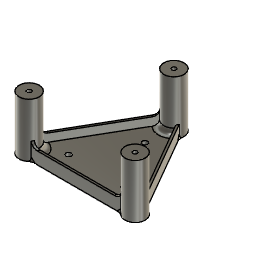
stevenson_spacer_bottom v5 (Autodesk Fusion 360 design; units mm, degrees)
Autodesk Fusion 360 part; units mm, degrees
sketch "Sketch1" plane through (0, 0, 0) normal (0, 0, 1) x (1, 0, 0)
  circle A0 centre (0, 0) radius 60 construction
  circle A1 centre (0, 0) radius 22.5 construction
  circle A2 centre (0, 0) radius 45.5 construction
  circle A3 centre (0, 45.5) radius 4.5
  circle A4 centre (-39.4042, -22.75) radius 4.5
  circle A5 centre (39.4042, -22.75) radius 4.5
  line L0 (0, 0) -> (0, 45.5) construction
  line L1 (0, 0) -> (39.4042, -22.75) construction
  line L2 (0, 0) -> (-39.4042, -22.75) construction
  circle A6 centre (-39.4042, -22.75) radius 2
  circle A7 centre (39.4042, -22.75) radius 2
  circle A8 centre (0, 45.5) radius 2
  line L3 (-43.3013, -20.5) -> (-3.8971, 47.75)
  line L4 (-39.4042, -27.25) -> (39.4042, -27.25)
  line L5 (3.8971, 47.75) -> (43.3013, -20.5)
  line L6 (-38.5819, -18.3258) -> (-3.4204, 42.5758)
  line L7 (3.4204, 42.5758) -> (38.5819, -18.3258)
  line L8 (-35.1615, -24.25) -> (35.1615, -24.25)
  dimension "d5" = 120
  dimension "d7" = 45
  dimension "d10" = 91
  dimension "d12" = 9
  dimension "d13" = 120
  dimension "d14" = 120
  dimension "d16" = 4
  dimension "d19" = 3
  dimension "d20" = 3
  dimension "d21" = 3
  constraint coincident A0.centre A1.centre
  constraint concentric A1 A2
  constraint coincident A2 A3.centre
  constraint coincident A2 A4.centre
  constraint coincident A2 A5.centre
  constraint equal A3 A5
  constraint equal A4 A5
  constraint coincident A3.centre L0.end
  constraint coincident A5.centre L1.end
  constraint coincident A4.centre L2.end
  constraint vertical A0.centre A3.centre
  constraint concentric A4 A6
  constraint concentric A5 A7
  constraint equal A7 A8
  constraint equal A6 A7
  constraint coincident A4 L3.start
  constraint coincident A3 L3.end
  constraint coincident A4 L4.start
  constraint coincident A5 L4.end
  constraint horizontal L4
  constraint coincident A3 L5.start
  constraint coincident A5 L5.end
  constraint equal L3 L5
  constraint equal L4 L5
  constraint tangent A3 L3
  constraint tangent A4 L3
  constraint tangent A5 L4
  constraint tangent A5 L5
  constraint coincident A4 L6.start
  constraint coincident A3 L6.end
  constraint coincident A3 L7.start
  constraint coincident A5 L7.end
  constraint coincident A4 L8.start
  constraint coincident A5 L8.end
  constraint horizontal L8
  constraint parallel L3 L6
  constraint parallel L5 L7
  measures "d5" diameter of A0
  measures "d7" diameter of A1
  measures "d10" diameter of A2
  measures "d12" diameter of A3
  measures "d13" angle of L0 L1
  measures "d14" angle of L1 L2
  measures "d16" diameter of A8
  measures "d19" distance of L3 L6
  measures "d20" distance of L4 L8
  measures "d21" distance of L5 L7
extrude "Extrude1" add sketch "Sketch1" along normal blind 3 makes body 1
extrude "Extrude2" add sketch "Sketch1" along normal blind 40 contours A3 | A5 | A4 bodies 1
sketch "Sketch3" plane through (0, 0, 40) normal (0, 0, 1) x (-1, 0, 0)
  circle A0 centre (39.4042, 22.75) radius 2
  circle A1 centre (39.4042, 22.75) radius 4.5
  circle A2 centre (39.4042, 22.75) radius 2.5
  circle A3 centre (-39.4042, 22.75) radius 2.5
  circle A4 centre (0, -45.5) radius 2.5
  dimension "d29" = 5
  dimension "d31" = 360
  constraint concentric A0 A2
  measures "d29" diameter of A2
extrude "Extrude3" cut sketch "Sketch3" against normal blind 5 contours A2 | A3 | A4 bodies 1
fillet "Fillet1" [no effect]
fillet "Fillet2" radius 5 3 edges at (35.507, -20.5, 3) (-35.507, -20.5, 3) (0, 41, 3) on bodies 1
sketch "Sketch5" plane through (0, 0, 0) normal (1, 0, 0) x (0, 1, 0)
  line L0 (60, 0) -> (-60, 0) construction
  line L1 (60, 40) -> (51.4977, 0)
  line L2 (51.4977, 0) -> (48.4307, 0)
  line L3 (48.4307, 0) -> (56.933, 40)
  line L4 (56.933, 40) -> (60, 40)
  line L5 (50, 40) -> (41, 40) construction
  line L6 (60, 40) -> (60, 0) construction
  dimension "d39" = 12
  dimension "d40" = 3
  constraint coincident L0 L1.end
  constraint coincident L0 L2.end
  constraint parallel L1 L3
  constraint parallel L0 L4
  constraint horizontal L3.end L5.start
  constraint vertical L0.start L1.start
  constraint coincident L0.start L6.end
  measures "d39" angle of L1 L6
  measures "d40" distance of L1 L3
revolve "Revolve1" add sketch "Sketch5" angle 360 about axis through (0, 0, 1.75) along (0, 0, 1) separate body makes body 2
sketch "Sketch7" plane through (0, 0, 40) normal (0, 0, 1) x (-1, 0, 0)
  circle A0 centre (0, 0) radius 56.933
  circle A1 centre (0, 0) radius 60
  line L0 (0, 0) -> (-30, -51.9615) construction
  line L1 (-23.7213, -55.5865) -> (-36.2787, -48.3365)
  line L2 (-36.2787, -48.3365) -> (-30.2212, -37.8446)
  line L3 (-30.2212, -37.8446) -> (-17.6638, -45.0946)
  line L4 (-17.6638, -45.0946) -> (-23.7213, -55.5865)
  circle A2 centre (0, 0) radius 48.4307 construction
  line L5 (0, 0) -> (0, -48.4307) construction
  dimension "d44" = 14.5
  dimension "d46" = 30
  constraint coincident A0.centre A1.centre
  constraint coincident A1 L0.end
  constraint midpoint L0.end L1
  constraint coincident L2.end A2
  constraint perpendicular L0 L1
  constraint perpendicular L1 L4
  constraint perpendicular L3 L4
  constraint perpendicular L2 L3
  constraint coincident A2 L5.end
  constraint vertical L5
  measures "d44" distance of L1.start L1.end
  measures "d46" angle of L0 L5
extrude "Extrude4" cut sketch "Sketch7" against normal blind 5.7 contours A0 L2 L3 L4 | A0 A1 L2 L4 picked at (-26.1412, -43.6629) picked at (-28.9605, -50.161) bodies 2
pattern_circular "C-Pattern1" count 6 over 360 about axis through (0, 0, 1.75) along (0, 0, 1) of "Extrude4"
chamfer "Chamfer2" distance 3.5 angle 45 12 edges at (-22.1182, 52.8098, 34.3) (22.1182, 52.8098, 34.3) (56.7937, 7.25, 34.3) (-56.7937, 7.25, 34.3) (-34.6755, -45.5598, 34.3) (34.6755, -45.5598, 34.3) (56.7937, -7.25, 34.3) (22.1182, -52.8098, 34.3) (-56.7937, -7.25, 34.3) (-34.6755, 45.5598, 34.3) (34.6755, 45.5598, 34.3) (-22.1182, -52.8098, 34.3) on bodies 2
sketch "Sketch8" plane through (0, 0, 0) normal (1, 0, 0) x (0, 1, 0)
  line L0 (90, 55) -> (-90, 55)
  line L1 (-90, 55) -> (-90, -30)
  line L2 (-90, -30) -> (90, -30)
  line L3 (90, -30) -> (90, 55)
  constraint horizontal L0
  constraint vertical L1
  constraint horizontal L2
  constraint vertical L3
sketch "Sketch9" plane through (0, 0, 0) normal (0, 0, -1) x (1, 0, 0)
  circle A0 centre (39.4042, 22.75) radius 2
  circle A1 centre (-39.4042, 22.75) radius 2
  arc A2 (43.3013, 20.5) -> (39.4042, 27.25) centre (39.4042, 22.75) ccw
  line L0 (39.4042, 27.25) -> (-39.4042, 27.25)
  arc A3 (-39.4042, 27.25) -> (-43.3013, 20.5) centre (-39.4042, 22.75) ccw
  line L1 (-43.3013, 20.5) -> (-3.8971, -47.75)
  arc A4 (-3.8971, -47.75) -> (3.8971, -47.75) centre (0, -45.5) ccw
  line L2 (3.8971, -47.75) -> (43.3013, 20.5)
  circle A5 centre (0, -45.5) radius 2
  circle A6 centre (0, -45.5) radius 2.5
  circle A7 centre (-39.4042, 22.75) radius 2.5
  circle A8 centre (39.4042, 22.75) radius 2.5
  dimension "d56" = 5
  constraint concentric A4 A6
  constraint concentric A1 A7
  constraint concentric A0 A8
  constraint equal A6 A7
  constraint equal A6 A8
  measures "d56" diameter of A6
extrude "Extrude6" cut sketch "Sketch9" against normal up to surface (33 mm away) contours A6 | A7 | A8 bodies 1
chamfer "Chamfer3" distance 0.5 angle 45 3 edges at (-41.735, -21.846, 33) (-2.3308, 46.404, 33) (37.0733, -21.846, 33) on bodies 1
sketch "Sketch10" plane through (0, 0, 40) normal (0, 0, 1) x (-1, 0, 0)
  circle A0 centre (0, -45.5) radius 2.5
  circle A1 centre (0, -45.5) radius 4.5
  arc A2 (-21.9561, -52.529) -> (21.9561, -52.529) centre (0, 0) ccw
  circle A3 centre (0, -45.5) radius 4.5
  circle A4 centre (0, -45.5) radius 2.5
  line L0 (21.9561, -52.529) -> (13.8983, -38.5725)
  line L1 (-21.9561, -52.529) -> (-13.8983, -38.5725)
  arc A5 (-13.8983, -38.5725) -> (13.8983, -38.5725) centre (0, 0) ccw
  line L2 (19.8231, -51.2316) -> (13.7644, -40.7375)
  line L3 (-19.8231, -51.2316) -> (-13.7644, -40.7375)
  arc A6 (-19.8231, -51.2316) -> (19.8231, -51.2316) centre (0, 0) ccw
  arc A7 (-5.8194, -42.6044) -> (5.8194, -42.6044) centre (0, -45.5) ccw
  arc A8 (-13.7644, -40.7375) -> (-5.8194, -42.6044) centre (0, 0) ccw
  arc A9 (5.8194, -42.6044) -> (13.7644, -40.7375) centre (0, 0) ccw
  arc A10 (-31.0451, -46.2717) -> (-24.5499, -50.0217) centre (0, 0) ccw construction
  arc A11 (24.5499, -50.0217) -> (31.0451, -46.2717) centre (0, 0) ccw construction
  line L4 (-27.8607, -48.2562) -> (0, 0) construction
  line L5 (0, 0) -> (27.8607, -48.2562) construction
  line L6 (0, -52) -> (0, -54.933) construction
  line L7 (1.0754, -51.9104) -> (1.0754, -54.9225)
  line L8 (-1.0754, -51.9104) -> (-1.0754, -54.9225)
  dimension "d70" = 2.1508
  constraint coincident A2.end L0.start
  constraint coincident A2.start L1.start
  constraint coincident L0.end A5.end
  constraint tangent A1 A5
  constraint concentric A1 A7
  constraint coincident A7.end A8
  constraint parallel L0 L2
  constraint concentric A5 A8
  constraint parallel L1 L3
  constraint concentric A2 A6
  constraint concentric A8 A9
  constraint midpoint A10 L4.start
  constraint coincident A2.centre A5.centre
  constraint midpoint A11 L5.end
  constraint parallel L0 L5
  constraint parallel L1 L4
  constraint midpoint A7 L6.start
  constraint midpoint A6 L6.end
  constraint vertical L6
  constraint coincident A7 L7.start
  constraint coincident A6 L7.end
  constraint vertical L7
  constraint coincident A7 L8.start
  constraint coincident A6 L8.end
  constraint parallel L6 L8
  constraint equal L7 L8
  measures "d70" distance of L7 L8
extrude "Extrude7" add sketch "Sketch10" against normal blind 1.2 contours A1 A3 | A2 L0 L1 A5 | A6 A7 L7 L8 bodies 2
pattern_circular "C-Pattern2" count 6 over 360 about axis through (0, 0, 1.75) along (0, 0, 1) of "Extrude7"
sketch "Sketch11" plane through (0, 0, 0) normal (0, 0, 1) x (1, 0, 0)
  circle A0 centre (0, 0) radius 68.9895
  constraint coincident A0.centre origin
extrude "Extrude8" cut sketch "Sketch11" along normal up to surface (31.9 mm away) bodies 2
sketch "Sketch12" plane through (0, 0, 0) normal (1, 0, 0) x (0, 1, 0)
  line L0 (50, 40) -> (41, 40) construction
  line L1 (50, 0) -> (47.75, 0) construction
  line L2 (50, 40) -> (50, 0)
  line L3 (50, 40) -> (53, 40)
  line L4 (53, 40) -> (50, 35.7156)
  line L5 (50, 4.2844) -> (53, 0)
  line L6 (53, 0) -> (50, 0)
  dimension "d71" = 35
  dimension "d72" = 35
  dimension "d73" = 3
  constraint coincident L0.start L2.start
  constraint coincident L1.start L2.end
  constraint perpendicular L2 L3
  constraint coincident L2 L4.end
  constraint coincident L2 L5.start
  constraint perpendicular L2 L6
  constraint equal L3 L6
  measures "d71" angle of L2 L4
  measures "d72" angle of L2 L5
  measures "d73" distance of L0.start L3.end
revolve "Revolve2" add sketch "Sketch12" angle 360 about axis through (0, 45.5, 40) along (0, 0, 1) bodies 1
fillet "Fillet3" radius 4 3 edges at (5.1962, 45.5, 3.2902) (0, 50, 4.2844) (-5.1962, 45.5, 3.2902) on bodies 1
pattern_circular "C-Pattern3" count 3 over 360 about axis through (0, 0, 1.75) along (0, 0, 1) of "Revolve2", "Fillet3"
sketch "Sketch14" plane through (0, 0, 40) normal (0, 0, 1) x (-1, 0, 0)
  circle A0 centre (0, -45.5) radius 7.5
  circle A1 centre (0, -45.5) radius 2.5
  circle A2 centre (0, -45.5) radius 2.5
  line L0 (2, -47) -> (-2, -47)
  dimension "d80" = 4
  constraint coincident A2 L0.start
  constraint coincident A2 L0.end
  constraint horizontal L0
  measures "d80" distance of L0.start L0.end
extrude "Extrude9" add sketch "Sketch14" against normal up to surface (40 mm away) contours A1 A2 L0 picked at (-0.6667, -47.4632) bodies 1
pattern_circular "C-Pattern4" count 3 over 360 about axis through (0, 0, 1.75) along (0, 0, 1) of "Extrude9"
ref_plane "WorkPlane1" through (0, 45.5, 45) normal (0, 0, 1) x (1, 0, 0)
sketch "Sketch15" plane through (0, 45.5, 45) normal (0, 0, 1) x (1, 0, 0)
  arc A0 (-2, 1.5) -> (2, 1.5) centre (0, 0) ccw
  line L0 (-2, 1.5) -> (2, 1.5)
  arc A1 (-1.8974, 1.3) -> (1.8974, 1.3) centre (0, 0) ccw
  line L1 (-1.8974, 1.3) -> (1.8974, 1.3)
  dimension "d88" = 0.2
extrude "Extrude10" add sketch "Sketch15" along normal blind 15 separate body contours A1 L1 makes body 3
sketch "Sketch16" plane through (0, 0, 40) normal (0, 0, 1) x (-1, 0, 0)
  circle A0 centre (0, -45.5) radius 7.5
  arc A1 (2, -47) -> (-2, -47) centre (0, -45.5) ccw
  line L0 (2, -47) -> (-2, -47)
extrude "Extrude11" add sketch "Sketch16" 2 faces at (-42.4352, -24.5, 40) (42.4352, -24.5, 40) along normal up to surface end surface through (7.4268, 44.4549, 0) normal (0, 0, 1) offset 0 on bodies 1 bodies 1
fillet "Fillet4" radius 4 2 edges at (0, 38, 3.4174) (0, 38, 3.4174) on bodies 1
fillet "Fillet4" radius 4 4 edges at (-32.909, -19, 3.4174) (-32.909, -19, 3.4174) (32.909, -19, 3.4174) (32.909, -19, 3.4174) on bodies 1
sketch "Sketch17" plane through (0, 0, 3) normal (0, 0, 1) x (-1, 0, 0)
  arc A0 (-38.0098, 11.3348) -> (-28.8212, 27.25) centre (-39.4042, 22.75) ccw
  line L0 (-38.0098, 11.3348) -> (-9.1886, -38.5848)
  arc A1 (9.1886, -38.5848) -> (-9.1886, -38.5848) centre (0, -45.5) ccw
  line L1 (9.1886, -38.5848) -> (38.0098, 11.3348)
  arc A2 (28.8212, 27.25) -> (38.0098, 11.3348) centre (39.4042, 22.75) ccw
  line L2 (28.8212, 27.25) -> (-28.8212, 27.25)
  circle A3 centre (0, -24) radius 2
  circle A4 centre (20.7846, 12) radius 2
  circle A5 centre (-20.7846, 12) radius 2
  point P0 (0, -34)
  dimension "d97" = 4
  dimension "d98" = 10
  dimension "d100" = 360
  constraint midpoint A1 P0
  constraint vertical origin A3.centre
  measures "d97" diameter of A3
  measures "d98" distance of A3.centre P0
extrude "Extrude12" cut sketch "Sketch17" against normal up to surface (3 mm away) contours A3 | A4 | A5 bodies 1
sketch "Sketch18" plane through (0, 0, 3) normal (0, 0, 1) x (-1, 0, 0)
  circle A0 centre (20.7846, 12) radius 2
  circle A1 centre (0, -24) radius 2
  circle A2 centre (-20.7846, 12) radius 2
  arc A3 (-38.0098, 11.3348) -> (-28.8212, 27.25) centre (-39.4042, 22.75) ccw
  line L0 (-38.0098, 11.3348) -> (-9.1886, -38.5848)
  arc A4 (9.1886, -38.5848) -> (-9.1886, -38.5848) centre (0, -45.5) ccw
  line L1 (9.1886, -38.5848) -> (38.0098, 11.3348)
  arc A5 (28.8212, 27.25) -> (38.0098, 11.3348) centre (39.4042, 22.75) ccw
  line L2 (28.8212, 27.25) -> (-28.8212, 27.25)
  line L3 (35, 25.65) -> (-34.8846, 25.65)
  line L4 (-34.8846, 25.65) -> (-35.6422, 27.25)
  line L5 (-35.6422, 27.25) -> (35, 27.25)
  line L6 (35, 27.25) -> (35, 25.65)
  line L7 (-39.7136, 17.4859) -> (-4.7713, -43.0359)
  line L8 (-5.7781, -44.492) -> (-41.0992, 16.6859)
  line L9 (-41.0992, 16.6859) -> (-39.7136, 17.4859)
  line L10 (-4.7713, -43.0359) -> (-5.7781, -44.492)
  line L11 (4.7136, -43.1359) -> (39.6558, 17.3859)
  line L12 (41.4203, 17.242) -> (6.0992, -43.9359)
  line L13 (6.0992, -43.9359) -> (4.7136, -43.1359)
  line L14 (39.6558, 17.3859) -> (41.4203, 17.242)
  dimension "d103" = 1.6
  dimension "d105" = 360
  constraint parallel L2 L3
  constraint parallel L2 L5
  constraint perpendicular L5 L6
  constraint collinear L2 L5
  measures "d103" distance of L3 L5
extrude "Extrude13" add sketch "Sketch18" along normal blind 6 contours A3 L7 L8 L9 | A3 L0 A4 L7 L8 | A4 L7 L8 L10 | A3 L3 L4 L5 | A3 A5 L2 L3 L5 | A5 L3 L5 L6 | A4 L1 A5 L11 L12 | A4 L11 L12 L13 | A5 L11 L12 L14 bodies 1
fillet "Fillet5" radius 4 5 edges at (-6.4826, 41.7283, 9) (-39.3791, -15.25, 9) (-32.8965, -26.4783, 9) (39.3791, -15.25, 9) (32.8965, -26.4783, 9) on bodies 1
sketch "Sketch19" plane through (0, 0, 0) normal (0, 0, -1) x (1, 0, 0)
  circle A0 centre (-20.7846, 12) radius 2
  circle A1 centre (0, -24) radius 2
  circle A2 centre (20.7846, 12) radius 2
  arc A3 (39.7032, 25.2321) -> (41.7032, 21.7679) centre (39.4042, 22.75) ccw
  line L0 (39.7032, 25.2321) -> (41.7032, 21.7679)
  spline S0 degree 3 poles (30.3991, 27.25) (31.2433, 27.25) (32.0954, 27.3887) (33.6181, 27.9075) (34.264, 28.2527) (34.7938, 28.6656) knots 0 0 0 0 0.253267 0.253267 0.483496 0.483496 0.483496 0.483496
  line L1 (30.3991, 27.25) -> (-30.3991, 27.25)
  spline S1 degree 3 poles (-34.7938, 28.6656) (-34.2696, 28.2571) (-33.6317, 27.9148) (-32.1116, 27.3913) (-31.2513, 27.25) (-30.3991, 27.25) knots 0 0 0 0 0.19935 0.19935 0.423274 0.423274 0.423274 0.423274
  arc A4 (-34.7938, 28.6656) -> (-42.222, 15.7995) centre (-39.4042, 22.75) ccw
  spline S2 degree 3 poles (-38.7987, 12.7014) (-39.2216, 13.4338) (-39.7689, 14.1035) (-40.9801, 15.1619) (-41.6008, 15.5476) (-42.222, 15.7995) knots 0 0 0 0 0.253712 0.253712 0.483453 0.483453 0.483453 0.483453
  line L2 (-38.7987, 12.7014) -> (-8.3996, -39.9514)
  spline S3 degree 3 poles (-7.4283, -44.4651) (-7.3365, -43.8062) (-7.3591, -43.0817) (-7.6664, -41.5035) (-7.974, -40.6887) (-8.3996, -39.9514) knots 0 0 0 0 0.199576 0.199576 0.423259 0.423259 0.423259 0.423259
  arc A5 (-7.4283, -44.4651) -> (7.4283, -44.4651) centre (0, -45.5) ccw
  spline S4 degree 3 poles (8.3996, -39.9514) (7.9768, -40.6838) (7.6705, -41.4926) (7.3595, -43.0707) (7.3358, -43.8012) (7.4283, -44.4651) knots 0 0 0 0 0.253712 0.253712 0.483453 0.483453 0.483453 0.483453
  line L3 (8.3996, -39.9514) -> (38.7987, 12.7014)
  spline S5 degree 3 poles (42.222, 15.7995) (41.6055, 15.5495) (40.9894, 15.1676) (39.7763, 14.1125) (39.2244, 13.4387) (38.7987, 12.7014) knots 0 0 0 0 0.199576 0.199576 0.423259 0.423259 0.423259 0.423259
  arc A6 (42.222, 15.7995) -> (34.7938, 28.6656) centre (39.4042, 22.75) ccw
  arc A7 (2, -47) -> (-2, -47) centre (0, -45.5) ccw
  line L4 (2, -47) -> (-2, -47)
  arc A8 (-41.7032, 21.7679) -> (-39.7032, 25.2321) centre (-39.4042, 22.75) ccw
  line L5 (-41.7032, 21.7679) -> (-39.7032, 25.2321)
  circle A9 centre (39.4042, 22.75) radius 1.4
  circle A10 centre (0, -45.5) radius 1.4
  circle A11 centre (-39.4042, 22.75) radius 1.4
  dimension "d111" = 2.8
  constraint concentric A3 A9
  constraint concentric A5 A10
  constraint concentric A4 A11
  constraint equal A9 A11
  constraint equal A9 A10
  measures "d111" diameter of A11
extrude "Extrude14" add sketch "Sketch19" against normal up to surface (32.5001 mm away) contours A3 L0 | A7 L4 | A8 L5 bodies 1
chamfer "Chamfer4" distance 0.4 distance2 3 3 edges at (-40.7094, -23.2563, 0) (38.0989, -23.2563, 0) (-1.3053, 44.9937, 0) measured on face at (-0.0498, 0.0863, 0) measured on face at (-0.0498, 0.0863, 0) measured on face at (-0.0498, 0.0863, 0) on bodies 1
sketch "Sketch20" plane through (0, 0, 0) normal (0, 0, -1) x (1, 0, 0)
  circle A0 centre (39.4042, 22.75) radius 1.8
  spline S0 degree 3 poles (30.3991, 27.25) (31.2433, 27.25) (32.0954, 27.3887) (33.6181, 27.9075) (34.264, 28.2527) (34.7938, 28.6656) knots 0 0 0 0 0.253267 0.253267 0.483496 0.483496 0.483496 0.483496
  line L0 (30.3991, 27.25) -> (-30.3991, 27.25)
  spline S1 degree 3 poles (-34.7938, 28.6656) (-34.2696, 28.2571) (-33.6317, 27.9148) (-32.1116, 27.3913) (-31.2513, 27.25) (-30.3991, 27.25) knots 0 0 0 0 0.19935 0.19935 0.423274 0.423274 0.423274 0.423274
  arc A1 (-34.7938, 28.6656) -> (-42.222, 15.7995) centre (-39.4042, 22.75) ccw
  spline S2 degree 3 poles (-38.7987, 12.7014) (-39.2216, 13.4338) (-39.7689, 14.1035) (-40.9801, 15.1619) (-41.6008, 15.5476) (-42.222, 15.7995) knots 0 0 0 0 0.253712 0.253712 0.483453 0.483453 0.483453 0.483453
  line L1 (-38.7987, 12.7014) -> (-8.3996, -39.9514)
  spline S3 degree 3 poles (-7.4283, -44.4651) (-7.3365, -43.8062) (-7.3591, -43.0817) (-7.6664, -41.5035) (-7.974, -40.6887) (-8.3996, -39.9514) knots 0 0 0 0 0.199576 0.199576 0.423259 0.423259 0.423259 0.423259
  arc A2 (-7.4283, -44.4651) -> (7.4283, -44.4651) centre (0, -45.5) ccw
  spline S4 degree 3 poles (8.3996, -39.9514) (7.9768, -40.6838) (7.6705, -41.4926) (7.3595, -43.0707) (7.3358, -43.8012) (7.4283, -44.4651) knots 0 0 0 0 0.253712 0.253712 0.483453 0.483453 0.483453 0.483453
  line L2 (8.3996, -39.9514) -> (38.7987, 12.7014)
  spline S5 degree 3 poles (42.222, 15.7995) (41.6055, 15.5495) (40.9894, 15.1676) (39.7763, 14.1125) (39.2244, 13.4387) (38.7987, 12.7014) knots 0 0 0 0 0.199576 0.199576 0.423259 0.423259 0.423259 0.423259
  arc A3 (42.222, 15.7995) -> (34.7938, 28.6656) centre (39.4042, 22.75) ccw
  circle A4 centre (20.7846, 12) radius 2
  circle A5 centre (0, -24) radius 2
  circle A6 centre (-20.7846, 12) radius 2
  circle A7 centre (-39.4042, 22.75) radius 1.8
  circle A8 centre (0, -45.5) radius 1.8
  circle A9 centre (-39.4042, 22.75) radius 5
  circle A10 centre (0, -45.5) radius 5
  circle A11 centre (39.4042, 22.75) radius 5
  dimension "d116" = 10
  constraint concentric A1 A9
  constraint concentric A2 A10
  constraint concentric A0 A11
  constraint equal A9 A11
  constraint equal A10 A11
  measures "d116" diameter of A11
extrude "Extrude15" cut sketch "Sketch20" against normal up to surface (40 mm away) contours A0 | A7 | A8 | A9 | A10 | A11 bodies 1
sketch "Sketch23" plane through (0, 0, 40) normal (0, 0, 1) x (-1, 0, 0)
  circle A0 centre (0, -45.5) radius 5
  circle A1 centre (0, -45.5) radius 7.5
  circle A2 centre (0, -45.5) radius 5
  circle A3 centre (0, -45.5) radius 1.6
  dimension "d119" = 3.2
  constraint concentric A0 A2
  constraint equal A0 A2
  constraint concentric A2 A3
  measures "d119" diameter of A3
extrude "Extrude16" add sketch "Sketch23" against normal blind 3 contours A0 A2 bodies 1
pattern_circular "C-Pattern5" count 3 over 360 about axis through (0, 0, 1.75) along (0, 0, 1) of "Extrude16"
sketch "Sketch25" plane through (0, 0, 37) normal (0, 0, -1) x (1, 0, 0)
  circle A0 centre (0, -45.5) radius 1.6
  circle A1 centre (0, -45.5) radius 5
  circle A2 centre (0, -45.5) radius 1.6
  constraint concentric A0 A2
  constraint equal A0 A2
extrude "Extrude17" add sketch "Sketch25" against normal blind 0.2 contours A0 A2 bodies 1
pattern_circular "C-Pattern6" count 3 over 360 about axis through (0, 0, 1.75) along (0, 0, 1) of "Extrude17"
extrude "Extrude5" [suppressed]
hidden bodies 2 3
equation "dishBase_D = 120 mm"
equation "dishLip_ID = 137 mm"
equation "dishLip_d = 7.2 mm"
equation "dish_H = 36.5 mm"
equation "d5 = dishBase_D"
equation "dishBase_smooth_D = 45 mm"
equation "d7 = dishBase_smooth_D"
equation "dishGroove_H = 5.5 mm"
equation "mount_D = dishBase_smooth_D + ( 2 * 23 ) * 1 mm"
equation "d10 = mount_D"
equation "column_D = dowel_D2 + 4 mm"
equation "d12 = column_D"
equation "dowel_D1 = 4 mm"
equation "d16 = dowel_D1"
equation "leg_W = 3 mm"
equation "d19 = leg_W"
equation "d20 = d19"
equation "d21 = d19"
equation "spacer_H = 19 mm"
equation "spacer_t = 2 mm"
equation "d24 = spacer_t * 3 / 2"
equation "dowel_D2 = 5 mm"
equation "d29 = dowel_D2"
equation "d32 = -dowel_H"
equation "dowel_H = 5 mm"
equation "d39 = 90 deg - 78 deg"
equation "dishGroove_W = 14.5 mm"
equation "d44 = dishGroove_W"
equation "clearance = 0.2 mm"
equation "d48 = -( dishGroove_H + clearance )"
equation "d56 = dowel_D2"
equation "d72 = d71"
equation "d88 = clearance"
equation "M4_D = 4 mm"
equation "M5_washer_D = 10 mm"
equation "d97 = M4_D"
equation "d98 = M5_washer_D"
equation "M3_D = 2.8 mm"
equation "d111 = M3_D"
equation "d114 = clearance * 2"
equation "d119 = M3_D + clearance * 2"
equation "d120 = -leg_W"
